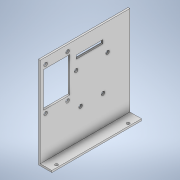
# Autodesk Inventor part: 板
Saved by Autodesk Inventor 2022.5 (Build 265521000, 521)
## iProperties
Created: 2025-01-08
Part Number: 板
Material: 常规
Document SubType Name: Modeling
Designer: Administrator
Density: 1 g/cm^3
Appearance: 默认
Mass: 20.2065 g
Surface Area: 217.189 cm^2
Volume: 20.2065 cm^3
Author: Administrator
Autodesk Inventor part; units mm, degrees
ref_plane "YZ Plane" through (0, 0, 0) normal (1, 0, 0) x (0, 1, 0)
ref_plane "XZ Plane" through (0, 0, 0) normal (0, 1, 0) x (-1, 0, 0)
ref_plane "XY Plane" through (0, 0, 0) normal (0, 0, 1) x (1, 0, 0)
sketch "草图1" plane through (0, 0, 0) normal (1, 0, 0) x (0, 1, 0)
  line L0 (0, 0) -> (100, 0)
  line L1 (100, 0) -> (100, -100)
  line L2 (100, -100) -> (0, -100)
  line L3 (0, -100) -> (0, 0)
  dimension "d0" = 100
  dimension "d1" = 100
  constraints: 8 end point, 2 parallel, 1 horizontal, 1 perpendicular
  measures "d0" distance of L1.end L2.end
  measures "d1" distance of L0.end L1.end
extrude "拉伸1" add sketch "草图1" along normal blind 2
sketch "草图2" plane through (0, 0, -100) normal (0, -1, 0) x (1, 0, 0)
  line L0 (0, 0) -> (0, 100) projected
  line L1 (0, 100) -> (15, 100)
  line L2 (15, 100) -> (15, 0)
  line L3 (15, 0) -> (0, 0)
  line L4 (0, 0) -> (0, 100)
  dimension "d30" = 15
  constraints: 8 end point, 2 parallel, 1 horizontal, 1 perpendicular
  measures "d30" distance of L0.end L1.end
extrude "拉伸2" add sketch "草图2" along normal blind 2
sketch "草图3" plane through (0, -2, -100) normal (0, -1, 0) x (1, 0, 0)
  circle A0 centre (12, 92) radius 1.6
  line L0 (0, 100) -> (0, 0) projected
  circle A1 centre (12, 12) radius 1.6
  line L1 (0, 0) -> (15, 0) projected
  dimension "d6" = 12
  dimension "d7" = 12
  dimension "d8" = 80
  dimension "d9" = 12
  dimension "d12" = 3.2
  dimension "d13" = 3.2
  constraints: 2 centre point
  measures "d6" distance from line of L0 A0.centre
  measures "d7" distance from line of L0 A1.centre
  measures "d8" distance of A0.centre A1.centre
  measures "d9" distance from line of L1 A1.centre
  measures "d12" diameter of A0
  measures "d13" diameter of A1
extrude "拉伸3" cut sketch "草图3" against normal blind 2
sketch "草图4" plane through (2, 0, 0) normal (1, 0, 0) x (0, 0, -1)
  line L0 (40, 85) -> (70, 85)
  line L1 (70, 85) -> (70, 81)
  line L2 (70, 81) -> (40, 81)
  line L3 (40, 81) -> (40, 85)
  line L4 (100, 100) -> (0, 100) projected
  line L5 (0, 100) -> (0, 0) projected
  circle A0 centre (40, 70) radius 2
  circle A1 centre (75, 70) radius 2
  circle A2 centre (70, 33) radius 2
  circle A3 centre (45, 33) radius 2
  point P0 (40, 83)
  point P1 (70, 83)
  dimension "d14" = 30
  dimension "d15" = 15
  dimension "d16" = 40
  dimension "d17" = 4
  dimension "d18" = 13
  dimension "d19" = 13
  dimension "d20" = 35
  dimension "d21" = 5
  dimension "d22" = 37
  dimension "d23" = 25
  dimension "d24" = 4
  dimension "d25" = 4
  dimension "d26" = 4
  dimension "d27" = 4
  constraints: 8 end point, 4 centre point, 2 midpoint, 2 parallel, 1 horizontal, 1 perpendicular
  measures "d14" distance of L0.start L0.end
  measures "d15" distance between parallel lines of L4 L0
  measures "d16" distance from line of L5 point (40, 83)
  measures "d17" distance between parallel lines of L0 L2
  measures "d18" distance of A0.centre point (40, 83)
  measures "d19" vertical distance of point (70, 83) A1.centre
  measures "d20" distance of A1.centre A0.centre
  measures "d21" horizontal distance of A1.centre point (70, 83)
  measures "d22" vertical distance of A2.centre A1.centre
  measures "d23" distance of A2.centre A3.centre
  measures "d24" diameter of A2
  measures "d25" diameter of A3
  measures "d26" diameter of A0
  measures "d27" diameter of A1
extrude "拉伸4" cut sketch "草图4" against normal blind 2
sketch "草图5" plane through (2, 0, 0) normal (1, 0, 0) x (0, 0, -1)
  circle A0 centre (6, 93) radius 2
  circle A1 centre (30.5, 93) radius 2
  circle A2 centre (6, 45.5) radius 2
  line L0 (100, 100) -> (0, 100) projected
  line L1 (0, 100) -> (0, 0) projected
  circle A3 centre (30.5, 45.5) radius 2
  dimension "d31" = 4
  dimension "d32" = 4
  dimension "d33" = 24.5
  dimension "d34" = 47.5
  dimension "d35" = 7
  dimension "d36" = 7
  dimension "d37" = 6
  dimension "d38" = 6
  dimension "d39" = 4
  dimension "d40" = 4
  constraints: 4 centre point
  measures "d31" diameter of A0
  measures "d32" diameter of A1
  measures "d33" distance of A0.centre A1.centre
  measures "d34" distance of A0.centre A2.centre
  measures "d35" distance from line of L0 A0.centre
  measures "d36" distance from line of L0 A1.centre
  measures "d37" distance from line of L1 A0.centre
  measures "d38" distance from line of L1 A2.centre
  measures "d39" diameter of A3
  measures "d40" diameter of A2
sketch "草图6" plane through (2, 0, 0) normal (1, 0, 0) x (0, 0, -1)
  line L0 (3.5741, 89.1195) -> (33.1877, 89.1195)
  line L1 (33.1877, 89.1195) -> (33.1877, 49.9441)
  line L2 (33.1877, 49.9441) -> (3.5741, 49.9441)
  line L3 (3.5741, 49.9441) -> (3.5741, 89.1195)
  point P0 (0, 0)
  constraints: 8 end point, 2 parallel, 1 horizontal, 1 perpendicular
extrude "拉伸5" cut sketch "草图6" against normal blind 2
extrude "拉伸6" cut sketch "草图5" against normal blind 2
